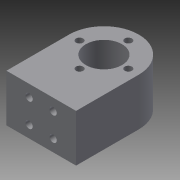
# Autodesk Inventor part: LimbAttachment
Saved by Autodesk Inventor 2015 (Build 190159000, 159)
## iProperties
Created: 2016-04-11
Part Number: LimbAttachment
Material: Generic
Document SubType Name: Modeling
Designer: Hatch
Density: 1 g/cm^3
Appearance: Default
Author: Hatch
Autodesk Inventor part; units mm, degrees
ref_plane "YZ Plane" through (0, 0, 0) normal (1, 0, 0) x (0, 1, 0)
ref_plane "XZ Plane" through (0, 0, 0) normal (0, 1, 0) x (-1, 0, 0)
ref_plane "XY Plane" through (0, 0, 0) normal (0, 0, 1) x (1, 0, 0)
sketch "Sketch1" plane through (0, 0, 0) normal (0, 1, 0) x (-1, 0, 0)
  circle A0 centre (7.5, 0) radius 13
  line L0 (-17.5, 45) -> (32.5, 45)
  line L1 (32.5, 45) -> (32.5, 0)
  line L2 (-17.5, 45) -> (-17.5, 0)
  arc A1 (-17.5, 0) -> (32.5, 0) centre (7.5, 0) ccw
  point P0 (0, 0)
  dimension "d1" = 26
  dimension "d6" = 50
  dimension "d29" = 45
  constraints: 6 end point, 2 centre point, 2 point on circle, 2 vertical, 1 coincident
  measures "d1" diameter of A0
  measures "d6" distance of L0.start L0.end
  measures "d29" distance of L0.start L2.end
extrude "Base" add sketch "Sketch1" along normal blind 34
sketch "Sketch3" plane through (0, 34, 0) normal (0, 1, 0) x (1, 0, 0)
  circle A0 centre (-7.5, 0) radius 13 projected
  line L0 (-7.5, 0) -> (-25, 0)
  line L1 (-25, 0) -> (10, 0)
  circle A1 centre (-25, 0) radius 2.6035
  point P0 (0, 0)
  dimension "d10" = 35
  dimension "d11" = 5.207
  constraints: 4 end point, 1 centre point, 1 coincident, 1 horizontal, 1 point on line
  measures "d10" distance of L0.end L1.end
  measures "d11" diameter of A1
extrude "Screw Hole" cut sketch "Sketch3" against normal through all contours A1
pattern_circular "Circular Pattern1" count 4 over 360 about axis through (-7.5, 0, 0) along (0, 1, 0) of "Screw Hole"
sketch "Sketch4" plane through (-32.5, 0, 45) normal (0, 0, 1) x (1, 0, 0)
  line L0 (0, 0) -> (0, 34) projected
  line L1 (0, 17) -> (50, 17)
  line L2 (50, 0) -> (50, 34) projected
  line L3 (25, 17) -> (25, 25.625)
  line L4 (25, 25.625) -> (33.5, 25.625)
  circle A0 centre (33.5, 25.625) radius 2.6035
  point P0 (32.5, 0)
  dimension "d17" = 8.625
  dimension "d18" = 8.5
  dimension "d19" = 5.207
  constraints: 6 end point, 3 midpoint, 1 centre point, 1 coincident, 1 horizontal, 1 vertical
  measures "d17" distance of L3.start L3.end
  measures "d18" distance of L3.end L4.end
  measures "d19" diameter of A0
extrude "Mount Holes" cut sketch "Sketch4" against normal blind 20
pattern_linear "Rectangular Pattern1" count 2 spacing 17 along (0, -1, 0) count 2 spacing 17.25 along (-1, 0, 0) of "Mount Holes"
body "Solid2"
